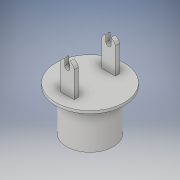
# Autodesk Inventor part: BaseComple
Saved by Autodesk Inventor 2019 (Build 230136000, 136)
## iProperties
Created: 2020-02-03
Part Number: BaseComple
Material: Generic
Document SubType Name: Modeling
Designer: Sergio
Density: 1 g/cm^3
Appearance: Default
Author: Sergio
Autodesk Inventor part; units mm, degrees
ref_plane "YZ Plane" through (0, 0, 0) normal (1, 0, 0) x (0, 1, 0)
ref_plane "XZ Plane" through (0, 0, 0) normal (0, 1, 0) x (-1, 0, 0)
sketch "Sketch1" plane through (0, 0, 0) normal (0, 1, 0) x (-1, 0, 0)
  circle A0 centre (0, 0) radius 25
  dimension "d12" = 50
  constraints: 1 centre point, 1 coincident
  measures "d12" diameter of A0
extrude "Extrusion1" add sketch "Sketch1" along normal blind 2
mirror "Mirror1" about plane through (0, 0, 0) normal (0, 0, 1)
ref_plane "Work Plane2" through (0, 0, 16.5) normal (0, 0, 1) x (1, 0, 0)
sketch "Sketch9" plane through (0, 0, 16.5) normal (0, 0, 1) x (1, 0, 0)
  line L0 (-5.099, 2) -> (5, 2)
  line L1 (5, 2) -> (5, 21)
  line L2 (-5.099, 20) -> (-5.099, 2)
  line L3 (0, -1.6) -> (0, 30.6) construction
  arc A0 (5, 21) -> (-5.099, 20) centre (0, 20) ccw
  circle A1 centre (0, 20) radius 1.9
  line L4 (25, 2) -> (-25, 2) projected
  dimension "d19" = 5
  dimension "d20" = 3.8
  dimension "d65" = 0
  dimension "d66" = 18
  constraints: 6 end point, 2 centre point, 2 point on circle, 1 coincident, 1 horizontal, 1 parallel, 1 perpendicular, 1 point on line
  measures "d19" distance between parallel lines of L3 L1
  measures "d20" diameter of A1
  measures "d65" distance between parallel lines of L4 L0
  measures "d66" distance from line of L0 A0.centre
extrude "Extrusion3" add sketch "Sketch9" against normal blind 3
sketch "Sketch20" plane through (0, 0, 16.5) normal (0, 0, 1) x (1, 0, 0)
  circle A0 centre (0, 20) radius 1.9 projected
  line L0 (-1.9, 20) -> (1.9, 20)
  line L1 (1.9, 20) -> (1.9, 25.4725)
  line L2 (1.9, 25.4725) -> (-1.9, 25.4725)
  line L3 (-1.9, 25.4725) -> (-1.9, 20)
  point P0 (0, 0)
  constraints: 8 end point, 2 parallel, 2 point on circle, 1 horizontal, 1 perpendicular
extrude "Extrusion14" cut sketch "Sketch20" against normal blind 3 contours A0 L3 L2 L1
mirror "Mirror5" about plane through (0, 0, 0) normal (0, 0, 1) of "Extrusion3", "Extrusion14"
sketch "Sketch21" plane through (0, 0, 0) normal (0, -1, 0) x (1, 0, 0)
  circle A0 centre (0, 0) radius 16.95
  dimension "d62" = 33.9
  constraints: 1 centre point, 1 coincident
  measures "d62" diameter of A0
extrude "Extrusion15" add sketch "Sketch21" along normal blind 30
ref_plane "Work Plane1" through (0, 0, 0) normal (0, 0, 1) x (1, 0, 0)
body "Solid1"
